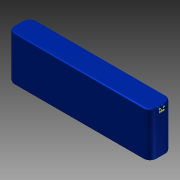
# Autodesk Inventor part: Battery
Saved by Autodesk Inventor 2011 SP1 (Build 150282100, 282)
## iProperties
Created: 2011-06-14
Part Number: Battery
Document SubType Name: Modeling
Designer: Andrew G. Meyer
Mass: 117.704 g
Surface Area: 179.745 cm^2
Volume: 117.704 cm^3
Density: 1 g/cm^3
Author: Andrew G. Meyer
Autodesk Inventor part; units mm, degrees
ref_plane "YZ Plane" through (0, 0, 0) normal (1, 0, 0) x (0, 1, 0)
ref_plane "XZ Plane" through (0, 0, 0) normal (0, 1, 0) x (-1, 0, 0)
ref_plane "XY Plane" through (0, 0, 0) normal (0, 0, 1) x (1, 0, 0)
sketch "Sketch1" plane through (0, 0, 0) normal (0, 0, 1) x (1, 0, 0)
  line L0 (-30.3593, 29.9629) -> (104.2607, 29.9629)
  line L1 (104.2607, 29.9629) -> (104.2607, -12.4551)
  line L2 (104.2607, -12.4551) -> (-30.3593, -12.4551)
  line L3 (-30.3593, -12.4551) -> (-30.3593, 29.9629)
  point P0 (0, 0)
  dimension "d0" = 42.418
  dimension "d1" = 134.62
  constraints: 8 end point, 2 parallel, 1 horizontal, 1 perpendicular
  measures "d0" distance of L2.end L0.start
  measures "d1" distance of L1.end L2.end
extrude "Extrusion1" add sketch "Sketch1" along normal blind 20.9042
sketch "Sketch2" plane through (104.2607, -12.4551, 0) normal (1, 0, 0) x (0, 0, -1)
  line L0 (-20.9042, 42.418) -> (-20.9042, 0) projected
  line L1 (0, 42.418) -> (0, 0) projected
  line L2 (0, 42.418) -> (-20.9042, 42.418) projected
  circle A0 centre (-12.3952, 40.4749) radius 1.9431
  circle A1 centre (-8.509, 40.4749) radius 1.9431
  line L3 (-12.3952, 40.4749) -> (-20.9042, 40.4749) construction
  line L4 (-8.509, 40.4749) -> (0, 40.4749) construction
  circle A2 centre (-10.4521, 37.7571) radius 0.7747
  circle A3 centre (-8.9027, 37.7571) radius 0.7747
  circle A4 centre (-12.0015, 37.7571) radius 0.7747
  line L5 (-10.4521, 42.418) -> (-10.4521, 37.7571) construction
  line L6 (-12.3952, 38.5318) -> (-8.509, 38.5318) construction
  line L7 (-12.0015, 37.7571) -> (-8.9027, 37.7571) construction
  point P0 (0, 12.4551)
  dimension "d4" = 3.8862
  dimension "d5" = 1.5494
  constraints: 10 end point, 4 equal radius, 3 centre point, 3 horizontal, 3 perpendicular, 2 midpoint, 2 parallel, 2 point on line, 2 vertical alignment, 1 collinear, 1 tangent, 4 other
  measures "d5" diameter of A4
extrude "Extrusion2" add sketch "Sketch2" along normal blind 0.254 contours A1 | A0 | A2 | A4 | A3
fillet "Fillet1" radius 6.35 4 edges at (104.2607, 8.7539, 20.9042) (104.2607, 8.7539, 0) (-30.3593, 8.7539, 0) (-30.3593, 8.7539, 20.9042)
fillet "Fillet2" radius 1.27 18 edges at (36.9507, 29.9629, 20.9042) (102.4008, 29.9629, 19.0443) (104.2607, 29.9629, 13.4747) (-28.4994, 29.9629, 19.0443) (-30.3593, 29.9629, 10.4521) (-28.4994, 29.9629, 1.8599) (36.9507, 29.9629, 0) (102.4008, 29.9629, 1.8599) (104.2607, 29.9629, 7.4295) (36.9507, -12.4551, 20.9042) (-28.4994, -12.4551, 19.0443) (-30.3593, -12.4551, 10.4521) (-28.4994, -12.4551, 1.8599) (36.9507, -12.4551, 0) (102.4008, -12.4551, 1.8599) (104.2607, -12.4551, 10.4521) (102.4008, -12.4551, 19.0443) (104.2607, 29.9629, 10.4521)
sketch "Sketch3" plane through (104.5147, 28.0198, 8.509) normal (1, 0, 0) x (0, 0, -1)
  circle A0 centre (0, 0) radius 1.9431 construction
  point P0 (-1.9431, 0)
  constraints: 1 horizontal alignment
sketch "Sketch4" plane through (104.5147, 28.0198, 12.3952) normal (1, 0, 0) x (0, 0, -1)
  circle A0 centre (0, 0) radius 1.9431 construction
  point P0 (1.9431, 0)
  constraints: 1 horizontal alignment
sketch "Sketch5" plane through (104.5147, 25.302, 12.0015) normal (1, 0, 0) x (0, 0, -1)
  circle A0 centre (0, 0) radius 0.7747 construction
  point P0 (0.7747, 0)
  constraints: 1 horizontal alignment
sketch "Sketch6" plane through (104.5147, -12.4551, 0) normal (1, 0, 0) x (0, 0, -1)
  arc A0 (-11.2268, 37.7571) -> (-9.6774, 37.7571) centre (-10.4521, 37.7571) ccw construction
sketch "Sketch7" plane through (104.5147, 25.302, 8.9027) normal (1, 0, 0) x (0, 0, -1)
  circle A0 centre (0, 0) radius 0.7747 construction
  point P0 (-0.7747, 0)
  constraints: 1 horizontal alignment
body "Solid1"
